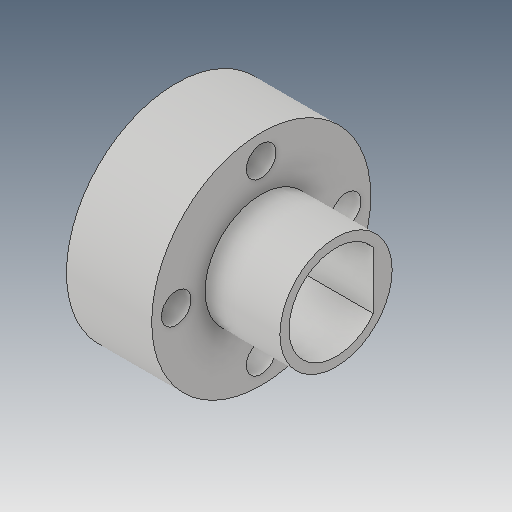
# Autodesk Inventor part: Our omiwheelinsert
Saved by Autodesk Inventor 2020 (Build 240168000, 168)
## iProperties
Created: 2019-09-23
Part Number: Our omiwheelinsert
Material: Generic
Document SubType Name: Modeling
Designer: ball
Density: 1 g/cm^3
Appearance: Default
Author: ball
Autodesk Inventor part; units mm, degrees
ref_plane "YZ Plane" through (0, 0, 0) normal (1, 0, 0) x (0, 1, 0)
ref_plane "XZ Plane" through (0, 0, 0) normal (0, 1, 0) x (-1, 0, 0)
ref_plane "XY Plane" through (0, 0, 0) normal (0, 0, 1) x (1, 0, 0)
sketch "Sketch1" plane through (0, 0, 0) normal (1, 0, 0) x (0, 1, 0)
  circle A0 centre (0, 0) radius 7.7343
  dimension "d0" = 15.4686
  constraints: 1 centre point, 1 coincident
  measures "d0" diameter of A0
extrude "Extrusion1" add sketch "Sketch1" along normal blind 6.0198
sketch "Sketch2" plane through (6.0198, 0, 0) normal (1, 0, 0) x (0, 0, -1)
  circle A0 centre (0, 0) radius 3.9624
  dimension "d3" = 7.9248
  constraints: 1 centre point, 1 coincident
  measures "d3" diameter of A0
extrude "Extrusion2" add sketch "Sketch2" along normal blind 5.2832
sketch "Sketch3" plane through (0, 0, 0) normal (-1, 0, 0) x (0, 0, 1)
  arc A0 (-2.6416, -2.0232) -> (-2.6416, 2.0232) centre (0, 0) ccw
  line L0 (-2.6416, -2.0232) -> (-2.6416, 2.0232)
  dimension "d6" = 6.6548
  constraints: 2 end point, 2 point on circle, 1 centre point, 1 coincident, 1 vertical
  measures "d6" diameter of A0
extrude "Extrusion3" cut sketch "Sketch3" against normal through all
sketch "Sketch4" plane through (0, 0, 0) normal (-1, 0, 0) x (0, 0, 1)
  circle A0 centre (0, 6) radius 1.05
  circle A1 centre (-6, 0) radius 1.05
  circle A2 centre (0, -6) radius 1.05
  circle A3 centre (6, 0) radius 1.05
  point P0 (0, 0)
  point P1 (0, 0)
  point P2 (0, 0)
  point P3 (0, 0)
  dimension "d12" = 2.1
  dimension "d13" = 6
  dimension "d14" = 0
  dimension "d17" = 360
  constraints: 4 centre point, 2 coincident, 11 other
  measures "d12" diameter of A0
  measures "d13" distance of A0.centre point (0, 0)
  measures "d14" horizontal distance of A0.centre point (0, 0)
extrude "Extrusion4" cut sketch "Sketch4" against normal through all
body "Solid1"
